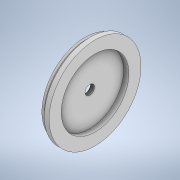
# Autodesk Inventor part: Крышка тих
Saved by Autodesk Inventor 2021 (Build 250183000, 183)
## iProperties
Created: 2023-04-26
Part Number: Крышка тих
Material: Типовые
Document SubType Name: Modeling
Designer: gdevc
Density: 1 g/cm^3
Appearance: По умолчанию
Mass: 49.2851 g
Surface Area: 189.776 cm^2
Volume: 49.2851 cm^3
Author: gdevc
Autodesk Inventor part; units mm, degrees
ref_plane "YZ Plane" through (0, 0, 0) normal (1, 0, 0) x (0, 1, 0)
ref_plane "XZ Plane" through (0, 0, 0) normal (0, 1, 0) x (-1, 0, 0)
ref_plane "XY Plane" through (0, 0, 0) normal (0, 0, 1) x (1, 0, 0)
sketch "Эскиз1" plane through (0, 0, 0) normal (0, 0, 1) x (1, 0, 0)
  line L0 (0, 0) -> (6.2046, 0)
  line L1 (0, 0) -> (0, 45)
  line L2 (0, 45) -> (2.55, 45)
  line L3 (2.55, 45) -> (3.05, 44.5)
  line L4 (3.05, 44.5) -> (5.55, 44.5)
  line L5 (5.55, 44.5) -> (5.55, 48)
  line L6 (5.55, 48) -> (10.55, 48)
  line L7 (10.55, 48) -> (10.55, 35.3814)
  line L8 (10.55, 35.3814) -> (5, 35.3814)
  line L9 (5, 35.3814) -> (5, 0)
  line L10 (0, 0) -> (5, 0)
  dimension "d0" = 45
  dimension "d1" = 0.5
  dimension "d2" = 90
  dimension "d3" = 10.55
  dimension "d4" = 5
  dimension "d6" = 3
  dimension "d7" = 2.5
  dimension "d8" = 5
  constraints: 22 end point, 6 perpendicular, 1 collinear, 1 horizontal, 1 parallel, 1 point on line, 1 vertical
  measures "d0" angle of L2 L3
  measures "d1" distance between parallel lines of L4 L2
  measures "d2" diameter of L2 L0
  measures "d3" distance between parallel lines of L7 L1
  measures "d4" distance between parallel lines of L7 L5
  measures "d6" distance between parallel lines of L2 L6
  measures "d7" distance of L3.end L4.end
  measures "d8" distance between parallel lines of L1 L9
revolve "Вращение1" add sketch "Эскиз1" angle 360 about axis through (0, 0, 0) along (1, 0, 0)
sketch "Эскиз2" plane through (0, 0, 0) normal (-1, 0, 0) x (0, 0, 1)
  circle A0 centre (0, 0) radius 5
  dimension "d10" = 10
  constraints: 1 centre point, 1 coincident
  measures "d10" diameter of A0
extrude "Выдавливание1" cut sketch "Эскиз2" against normal through all
thread "Резьба1" size "M10x1.5" class "6H" standard "ANSI Metric M Profile" length 10
chamfer "Фаска1" distance 1 angle 45 1 edges at (0, 0, -5)
